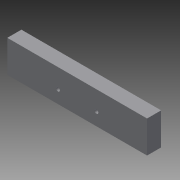
# Autodesk Inventor part: Xtion_Flame_1
Saved by Autodesk Inventor 2013 (Build 170138000, 138)
## iProperties
Created: 2014-04-24
Part Number: Xtion_Flame_1
Material: 一般
Document SubType Name: Modeling
Designer: andou
Density: 1 g/cm^3
Author: andou
Autodesk Inventor part; units mm, degrees
ref_plane "YZ Plane" through (0, 0, 0) normal (1, 0, 0) x (0, 1, 0)
ref_plane "XZ Plane" through (0, 0, 0) normal (0, 1, 0) x (-1, 0, 0)
ref_plane "XY Plane" through (0, 0, 0) normal (0, 0, 1) x (1, 0, 0)
sketch "スケッチ1" plane through (0, 0, 0) normal (0, 0, 1) x (1, 0, 0)
  line L0 (-54.5, 10) -> (54.5, 10)
  line L1 (54.5, 10) -> (54.5, -10)
  line L2 (54.5, -10) -> (-54.5, -10)
  line L3 (-54.5, -10) -> (-54.5, 10)
  line L4 (-54.5, 1) -> (-16.75, 1)
  line L5 (54.5, 1) -> (16.75, 1)
  arc A0 (-16.75, 1) -> (-11.75, 6) centre (-16.75, 6) ccw
  arc A1 (11.75, 6) -> (16.75, 1) centre (16.75, 6) ccw
  line L6 (-11.75, 6) -> (-11.75, 10)
  line L7 (11.75, 6) -> (11.75, 10)
  point P0 (0, 0)
  dimension "d0" = 109
  dimension "d2" = 54.5
  dimension "d3" = 20
  dimension "d4" = 10
  dimension "d5" = 11
  dimension "d6" = 11
  dimension "d11" = 5
  dimension "d14" = 10
  dimension "d23" = 23.5
  dimension "d25" = 5
  dimension "d28" = 16.75
  constraints: 16 end point, 4 perpendicular, 4 point on circle, 4 point on line, 3 equal length, 2 centre point, 2 tangent, 1 equal radius, 1 horizontal
  measures "d0" distance of L0.start L0.end
  measures "d2" distance from line of point (0, 0) L3
  measures "d3" distance between parallel lines of L0 L2
  measures "d4" distance from line of point (0, 0) L2
  measures "d5" distance between parallel lines of L2 L4
  measures "d6" distance between parallel lines of L5 L2
  measures "d11" distance from line of A0.centre L4
  measures "d14" diameter of A1
  measures "d23" distance between parallel lines of L7 L6
  measures "d25" distance from line of L5 A1.centre
  measures "d28" horizontal distance of point (0, 0) A0.centre
extrude "押し出し1" add sketch "スケッチ1" along normal blind 26 contours L0 L7 A1 L5 L1 L2 L3 L4 A0 L6
sketch "スケッチ4" plane through (0, 0, 0) normal (0, 0, -1) x (-1, 0, 0)
  line L0 (-54.5, -10) -> (-54.5, 1) projected
  line L1 (54.5, -10) -> (-54.5, -10) projected
  line L2 (54.5, 1) -> (54.5, -10) projected
  arc A0 (11.75, 6) -> (16.75, 1) centre (16.75, 6) ccw projected
  line L3 (-11.75, 10) -> (11.75, 10) projected
  line L4 (-11.75, 6) -> (-11.75, 10) projected
  arc A1 (-16.75, 1) -> (-11.75, 6) centre (-16.75, 6) ccw projected
  line L5 (-54.5, 1) -> (-16.75, 1) projected
  line L6 (-16.75, -2) -> (-51.5, -2)
  line L7 (-51.5, -2) -> (-51.5, -7)
  line L8 (-51.5, -7) -> (51.5, -7)
  line L9 (51.5, -7) -> (51.5, -2)
  line L10 (-8.75, 6) -> (-8.75, 10)
  line L11 (8.75, 10) -> (8.75, 6)
  arc A2 (-16.75, -2) -> (-8.75, 6) centre (-16.75, 6) ccw
  arc A3 (8.75, 6) -> (16.75, -2) centre (16.75, 6) ccw
  line L12 (16.75, -2) -> (51.5, -2)
  point P0 (0, 0)
  dimension "d55" = 16
  dimension "d59" = 17.5
  dimension "d60" = 3
  dimension "d61" = 3
  dimension "d62" = 3
  dimension "d63" = 3
  dimension "d64" = 3
  constraints: 14 end point, 5 parallel, 4 point on circle, 3 point on line, 2 centre point, 2 coincident, 2 perpendicular, 1 equal radius, 1 tangent
  measures "d55" diameter of A2
  measures "d59" distance between parallel lines of L11 L10
  measures "d60" distance between parallel lines of L4 L10
  measures "d61" distance between parallel lines of L5 L6
  measures "d62" distance between parallel lines of L1 L8
  measures "d63" distance between parallel lines of L0 L7
  measures "d64" distance between parallel lines of L2 L9
extrude "押し出し3" cut sketch "スケッチ4" against normal blind 24
sketch "スケッチ5" plane through (0, 0, 24) normal (0, 0, -1) x (-1, 0, 0)
  arc A0 (8.75, 6) -> (16.75, -2) centre (16.75, 6) ccw projected
  line L0 (8.75, 10) -> (8.75, 6) projected
  line L1 (-8.75, 10) -> (8.75, 10) projected
  line L2 (-8.75, 6) -> (-8.75, 10) projected
  arc A1 (-16.75, -2) -> (-8.75, 6) centre (-16.75, 6) ccw projected
  line L3 (-51.5, -2) -> (-16.75, -2) projected
  line L4 (16.75, -2) -> (-16.75, -2)
  point P0 (0, 0)
  constraints: 2 end point, 2 tangent, 1 collinear, 1 point on circle
extrude "押し出し4" add sketch "スケッチ5" along normal blind 10
sketch "スケッチ6" plane through (54.5, -10, 0) normal (1, 0, 0) x (0, 0, -1)
  line L0 (0, 0) -> (0, 11) projected
  line L1 (0, 11) -> (-26, 11) projected
  arc A0 (-26, 11) -> (-16, 20) centre (-29.9689, 25.4654) ccw
  line L2 (-26, 11) -> (-26, 20)
  line L3 (-26, 20) -> (-16, 20)
  point P0 (0, 10)
  dimension "d70" = 16
  dimension "d71" = 9
  dimension "d72" = 15
  constraints: 4 end point, 2 point on circle, 1 centre point, 1 parallel, 1 perpendicular
  measures "d70" distance from line of L0 L3.end
  measures "d71" distance from line of L1 L3.end
  measures "d72" radius of A0
extrude "押し出し5" cut sketch "スケッチ6" against normal blind 109
sketch "スケッチ7" plane through (-54.5, -10, 0) normal (0, -1, 0) x (1, 0, 0)
  line L0 (0, 0) -> (109, 0) projected
  circle A0 centre (39.5, 11) radius 1.5
  circle A1 centre (69.5, 11) radius 1.5
  point P0 (54.5, 0)
  dimension "d78" = 30
  dimension "d79" = 15
  dimension "d82" = 11
  dimension "d83" = 11
  dimension "d92" = 3
  constraints: 2 centre point, 1 equal radius
  measures "d78" distance of A1.centre A0.centre
  measures "d79" horizontal distance of A1.centre point (54.5, 0)
  measures "d82" distance from line of A1.centre L0
  measures "d83" distance from line of L0 A0.centre
  measures "d92" diameter of A1
hole "穴1" at (15, -10, 11) at (-15, -10, 11) direction (0, 1, 0) diameter 3 depth 4 tip angle 118
lip "リップ3" kind groove height 1 width 1 edges at (-54.5, -4.5, 0) (-35.625, 1, 0) (-13.2145, 2.4645, 0) (-11.75, 8, 0) (0, -10, 0) (35.625, 1, 0) (13.2145, 2.4645, 0) (11.75, 8, 0) (54.5, -4.5, 0) guide face at (17.1667, -9, 0)
